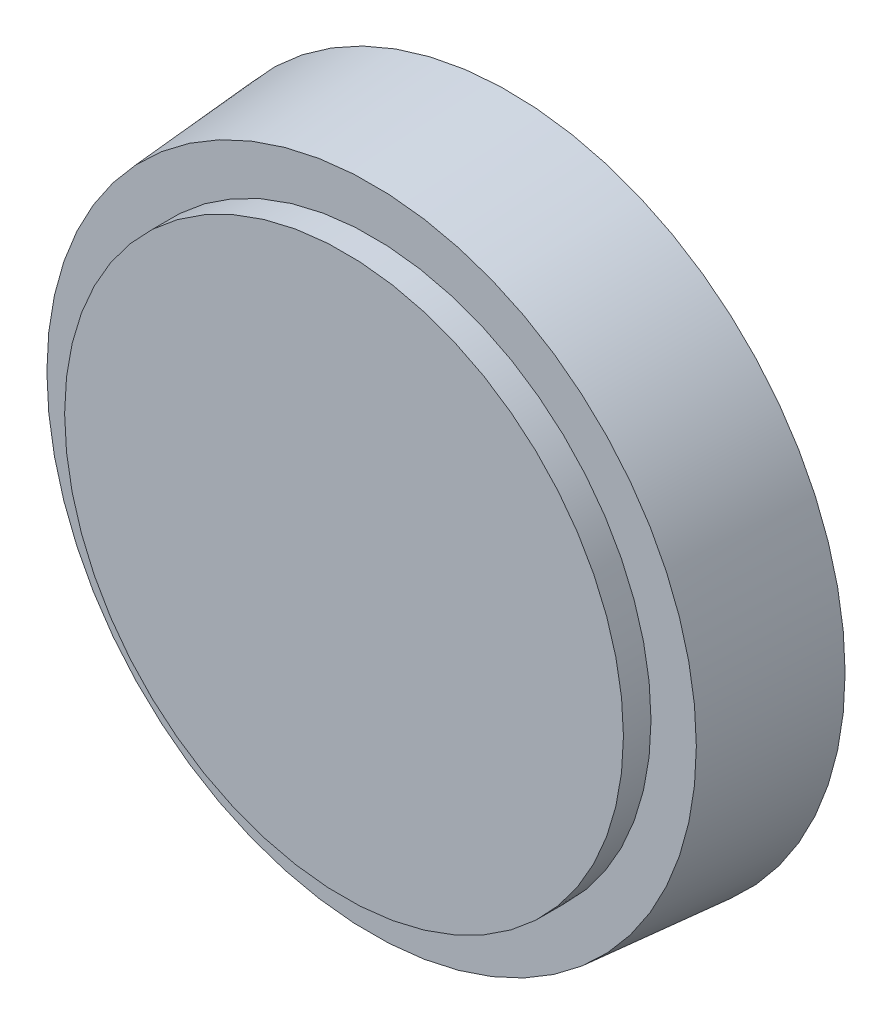
# Autodesk Inventor part: CUP
Saved by Autodesk Inventor 2022 (Build 260153070, 153G)
## iProperties
Created: 2021-11-19
Part Number: CUP
Material: Типовые
Document SubType Name: Modeling
Designer: kalugin_a
Density: 1 g/cm^3
Appearance: Резина — черная — версия 1.1
Author: kalugin_a
Autodesk Inventor part; units mm, degrees
ref_plane "YZ Plane" through (0, 0, 0) normal (1, 0, 0) x (0, 1, 0)
ref_plane "XZ Plane" through (0, 0, 0) normal (0, 1, 0) x (-1, 0, 0)
ref_plane "XY Plane" through (0, 0, 0) normal (0, 0, 1) x (1, 0, 0)
sketch "Эскиз2" plane through (0, 0, 0) normal (0, 0, 1) x (1, 0, 0)
  circle A0 centre (0, 0) radius 36.5
  circle A1 centre (0, 0) radius 32.0179
  dimension "d2" = 73
  constraints: 2 centre point, 2 coincident
  measures "d2" diameter of A0
extrude "Выдавливание1" add sketch "Эскиз2" along normal blind 15 contours A0 | A1
draft "НаклГрань1" angle 4.5 pull direction (0, 0, 1) faces at (36.3902, -2.8285, 10) fixed edges at (-36.5, 0, 0)
shell "Оболочка1" thickness 2 removed faces 1 at (4.5012, 0.5261, 0)
sketch "Эскиз3" plane through (0, 0, 15) normal (0, 0, 1) x (1, 0, 0)
  circle A0 centre (0, 0) radius 30.3888
  constraints: 1 centre point, 1 coincident
extrude "Выдавливание2" add sketch "Эскиз3" along normal blind 3
